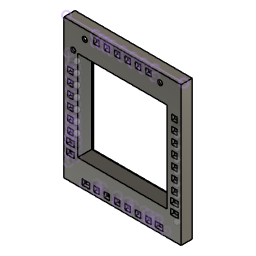
AH64-Iteration 6 v4 (Autodesk Fusion 360 design; units mm, degrees)
Autodesk Fusion 360 part; units mm, degrees
note: some values were not read from the file. Set by a fixed rule: which sketch regions a step uses.
(part 1 of 2)
sketch "Main Bezel" plane through (0, 0, 0) normal (0, 1, 0) x (1, 0, 0)
  line L0 (-54.051, 54.555) -> (-54.051, -54.555)
  line L1 (84.051, -99.755) -> (84.051, 99.755)
  line L2 (54.051, 54.555) -> (-54.051, 54.555)
  line L3 (-84.051, -99.755) -> (84.051, -99.755)
  line L4 (-54.051, -54.555) -> (54.051, -54.555)
  line L5 (-84.051, 99.755) -> (-84.051, -99.755)
  line L6 (84.051, 99.755) -> (-84.051, 99.755)
  line L7 (54.051, -54.555) -> (54.051, 54.555)
  point P0 (-27.075, -27.8271)
  dimension "d1" = 108.102
  dimension "d2" = 45.2
  dimension "d3" = 45.2
  dimension "d4" = 30
  dimension "d5" = 30
  dimension "d6" = 199.51
  dimension "d7" = 168.102
  dimension "d8" = 54.051
  dimension "d10" = 54.555
  dimension "d11" = 54.555
  dimension "d12" = 54.051
  constraint horizontal L4
  constraint vertical L7
  constraint horizontal L2
  constraint vertical L0
  constraint horizontal L3
  constraint vertical L1
  constraint horizontal L6
  constraint vertical L5
  measures "d1" distance of L0.end L4.end
  measures "d2" distance of L2 L6
  measures "d3" distance of L3 L4
  measures "d4" distance of L1 L7
  measures "d5" distance of L0 L5
  measures "d6" distance of L1.end L1.start
  measures "d7" distance of L3.start L1.start
  measures "d8" distance of origin L7
  measures "d10" distance of origin L4
  measures "d11" distance of origin L2
  measures "d12" distance of origin L0
extrude "Extrude1" add sketch "Main Bezel" along normal blind 16
sketch "LCD and Switch Insets" plane through (0, 16, 0) normal (0, 1, 0) x (-1, 0, 0)
  line L0 (-54.051, -54.555) -> (-54.051, 54.555)
  line L1 (-54.051, 54.555) -> (54.051, 54.555)
  line L2 (54.051, 54.555) -> (54.051, -54.555)
  line L3 (54.051, -54.555) -> (-54.051, -54.555)
  line L4 (-84.051, -99.755) -> (84.051, -99.755)
  line L5 (84.051, -99.755) -> (84.051, 99.755)
  line L6 (84.051, 99.755) -> (-84.051, 99.755)
  line L7 (-84.051, 99.755) -> (-84.051, -99.755)
  line L8 (-62.651, 73.5) -> (57.349, 73.5)
  line L9 (57.349, 73.5) -> (57.349, -81.5)
  line L10 (-62.651, -58.885) -> (-66.051, -58.885)
  line L11 (-66.051, -58.885) -> (-66.051, -8.885)
  line L12 (-66.051, -8.885) -> (-62.651, -8.885)
  line L13 (-52.651, -81.5) -> (-52.651, -84.7)
  line L14 (-52.651, -84.7) -> (-62.4877, -84.7)
  line L15 (-62.4877, -84.7) -> (-62.4877, -79.7)
  line L16 (-62.651, 73.5) -> (-62.651, -8.885)
  line L17 (-62.651, -58.885) -> (-62.4877, -79.7)
  line L18 (-52.651, -81.5) -> (57.349, -81.5)
  line L19 (-81.051, 62.605) -> (-68.051, 62.605)
  line L20 (-68.051, 62.605) -> (-68.051, -86.395)
  line L21 (-68.051, -86.395) -> (-81.051, -86.395)
  line L22 (-81.051, -86.395) -> (-81.051, 62.605)
  line L23 (68.051, 55.005) -> (81.051, 55.005)
  line L24 (81.051, 55.005) -> (81.051, -80.995)
  line L25 (81.051, -80.995) -> (68.051, -80.995)
  line L26 (68.051, -80.995) -> (68.051, 55.005)
  line L27 (-42.501, 96.755) -> (42.499, 96.755)
  line L28 (42.499, 96.755) -> (42.499, 86.755)
  line L29 (42.499, 86.755) -> (-42.501, 86.755)
  line L30 (-42.501, 86.755) -> (-42.501, 96.755)
  line L31 (-58.499, -86.755) -> (58.501, -86.755)
  line L32 (58.501, -86.755) -> (58.501, -96.755)
  line L33 (58.501, -96.755) -> (-58.499, -96.755)
  line L34 (-58.499, -96.755) -> (-58.499, -86.755)
  dimension "d15" = 120
  dimension "d18" = 3.298
  dimension "d19" = 18.945
  dimension "d21" = 3.4
  dimension "d22" = 50
  dimension "d23" = 10
  dimension "d24" = 5
  dimension "d25" = 13
  dimension "d27" = 37.15
  dimension "d28" = 3
  dimension "d29" = 13
  dimension "d30" = 136
  dimension "d31" = 3
  dimension "d32" = 44.75
  dimension "d33" = 85
  dimension "d34" = 10
  dimension "d35" = 3
  dimension "d36" = 41.55
  dimension "d37" = 117
  dimension "d38" = 10
  dimension "d39" = 3
  dimension "d40" = 25.55
  dimension "d108" = 149
  dimension "d109" = 13
  dimension "d170" = 3.2
  constraint horizontal L8
  constraint vertical L9
  constraint horizontal L10
  constraint vertical L11
  constraint horizontal L12
  constraint vertical L13
  constraint horizontal L14
  constraint vertical L15
  constraint perpendicular L12 L16
  constraint perpendicular L9 L18
  constraint horizontal L19
  constraint vertical L20
  constraint horizontal L21
  constraint vertical L22
  constraint horizontal L23
  constraint vertical L24
  constraint horizontal L25
  constraint vertical L26
  constraint horizontal L27
  constraint vertical L28
  constraint horizontal L29
  constraint vertical L30
  constraint horizontal L31
  constraint vertical L32
  constraint horizontal L33
  constraint vertical L34
  measures "d15" distance of L8.start L8.end
  measures "d18" distance of L2 L9
  measures "d19" distance of L1 L8
  measures "d21" distance of L10.start L10.end
  measures "d22" distance of L10.start L12.end
  measures "d23" distance of L15.end L13.start
  measures "d24" distance of L15.end L14.end
  measures "d25" distance of L19.start L19.end
  measures "d27" distance of L6 L19
  measures "d28" distance of L7 L22
  measures "d29" distance of L23.start L23.end
  measures "d30" distance of L23.start L25.end
  measures "d31" distance of L5 L24
  measures "d32" distance of L6 L23
  measures "d33" distance of L27.start L27.end
  measures "d34" distance of L27.start L29.end
  measures "d35" distance of L6 L27
  measures "d36" distance of L7 L30
  measures "d37" distance of L31.start L31.end
  measures "d38" distance of L31.start L33.end
  measures "d39" distance of L4 L33
  measures "d40" distance of L5 L32
  measures "d108" distance of L19.start L21.end
  measures "d109" distance of L20.end L21.end
  measures "d170" distance of L13.start L13.end
extrude "Extrude2" cut sketch "LCD and Switch Insets" against normal blind 5 contours L8 L9 L10 L11 L12 L13 L14 L15 L16 L17 L18
extrude "Extrude3" cut sketch "LCD and Switch Insets" against normal blind 12 contours L19 L20 L21 L22 | L23 L24 L25 L26 | L27 L28 L29 L30 | L31 L32 L33 L34
sketch "Button Holes" plane through (0, 16, 0) normal (0, 1, 0) x (-1, 0, 0)
  line L0 (-54.051, 54.5551) -> (-84.051, 54.5551) construction
  line L1 (-78.351, 41.5551) -> (-70.751, 41.5551)
  line L2 (-70.751, 41.5551) -> (-70.751, 33.9551)
  line L3 (-70.751, 33.9551) -> (-78.351, 33.9551)
  line L4 (-78.351, 33.9551) -> (-78.351, 41.5551)
  line L5 (-81.051, 62.605) -> (-68.051, 62.605)
  line L6 (-84.051, 99.755) -> (-84.051, -99.755)
  line L7 (-68.051, 62.605) -> (-68.051, -86.395)
  line L8 (-81.051, -86.395) -> (-81.051, 62.605)
  line L9 (84.051, 99.755) -> (-84.051, 99.755)
  line L10 (-78.351, 56.6551) -> (-70.751, 56.6551)
  line L11 (-70.751, 56.6551) -> (-70.751, 49.0551)
  line L12 (-70.751, 49.0551) -> (-78.351, 49.0551)
  line L13 (-78.351, 49.0551) -> (-78.351, 56.6551)
  line L14 (-78.351, -33.9474) -> (-70.751, -33.9474)
  line L15 (-70.751, -33.9474) -> (-70.751, -41.5474)
  line L16 (-70.751, -41.5474) -> (-78.351, -41.5474)
  line L17 (-78.351, -41.5474) -> (-78.351, -33.9474)
  line L18 (-54.051, -54.5474) -> (-84.051, -54.5474) construction
  line L19 (-84.051, -99.755) -> (84.051, -99.755)
  line L20 (-70.751, -26.4474) -> (-78.351, -26.4474)
  line L21 (-78.351, -26.4474) -> (-78.351, -18.8474)
  line L22 (-78.351, -18.8474) -> (-70.751, -18.8474)
  line L23 (-70.751, -18.8474) -> (-70.751, -26.4474)
  line L24 (-70.751, -11.3474) -> (-78.351, -11.3474)
  line L25 (-78.351, -11.3474) -> (-78.351, -3.7474)
  line L26 (-78.351, -3.7474) -> (-70.751, -3.7474)
  line L27 (-70.751, -3.7474) -> (-70.751, -11.3474)
  line L28 (-70.751, 3.7526) -> (-78.351, 3.7526)
  line L29 (-78.351, 3.7526) -> (-78.351, 11.3526)
  line L30 (-78.351, 11.3526) -> (-70.751, 11.3526)
  line L31 (-70.751, 11.3526) -> (-70.751, 3.7526)
  line L32 (-70.751, 18.8526) -> (-78.351, 18.8526)
  line L33 (-78.351, 18.8526) -> (-78.351, 26.4526)
  line L34 (-78.351, 26.4526) -> (-70.751, 26.4526)
  line L35 (-70.751, 26.4526) -> (-70.751, 18.8526)
  line L36 (-79.851, -47.5474) -> (-69.251, -47.5474)
  line L37 (-69.251, -47.5474) -> (-69.251, -55.1474)
  line L38 (-69.251, -55.1474) -> (-79.851, -55.1474)
  line L39 (-79.851, -55.1474) -> (-79.851, -47.5474)
  line L40 (-79.851, -61.1474) -> (-69.251, -61.1474)
  line L41 (-69.251, -61.1474) -> (-69.251, -68.7474)
  line L42 (-69.251, -68.7474) -> (-79.851, -68.7474)
  line L43 (-79.851, -68.7474) -> (-79.851, -61.1474)
  line L44 (78.351, 33.9551) -> (70.751, 33.9551)
  line L45 (70.751, 33.9551) -> (70.751, 41.5551)
  line L46 (70.751, 41.5551) -> (78.351, 41.5551)
  line L47 (78.351, 41.5551) -> (78.351, 33.9551)
  line L48 (70.751, 18.8526) -> (70.751, 26.4526)
  line L49 (70.751, 26.4526) -> (78.351, 26.4526)
  line L50 (78.351, 18.8526) -> (70.751, 18.8526)
  line L51 (78.351, 26.4526) -> (78.351, 18.8526)
  line L52 (70.751, 3.7526) -> (70.751, 11.3526)
  line L53 (70.751, 11.3526) -> (78.351, 11.3526)
  line L54 (78.351, 3.7526) -> (70.751, 3.7526)
  line L55 (78.351, 11.3526) -> (78.351, 3.7526)
  line L56 (70.751, -11.3474) -> (70.751, -3.7474)
  line L57 (70.751, -3.7474) -> (78.351, -3.7474)
  line L58 (78.351, -11.3474) -> (70.751, -11.3474)
  line L59 (78.351, -3.7474) -> (78.351, -11.3474)
  line L60 (70.751, -26.4474) -> (70.751, -18.8474)
  line L61 (70.751, -18.8474) -> (78.351, -18.8474)
  line L62 (78.351, -26.4474) -> (70.751, -26.4474)
  line L63 (78.351, -18.8474) -> (78.351, -26.4474)
  line L64 (70.751, -41.5474) -> (70.751, -33.9474)
  line L65 (70.751, -33.9474) -> (78.351, -33.9474)
  line L66 (78.351, -41.5474) -> (70.751, -41.5474)
  line L67 (78.351, -33.9474) -> (78.351, -41.5474)
  line L68 (84.051, -99.755) -> (84.051, 99.755)
  line L69 (68.051, -80.995) -> (68.051, 55.005)
  line L70 (69.251, -68.7474) -> (69.251, -61.1474)
  line L71 (69.251, -61.1474) -> (79.851, -61.1474)
  line L72 (79.851, -61.1474) -> (79.851, -68.7474)
  line L73 (79.851, -68.7474) -> (69.251, -68.7474)
  line L74 (79.851, -55.1474) -> (69.251, -55.1474)
  line L75 (69.251, -55.1474) -> (69.251, -47.5474)
  line L76 (79.851, -47.5474) -> (79.851, -55.1474)
  line L77 (69.251, -47.5474) -> (79.851, -47.5474)
  line L78 (-54.051, -54.5474) -> (-54.051, -99.755) construction
  line L79 (-41.051, -87.955) -> (-33.451, -87.955)
  line L80 (-33.451, -87.955) -> (-33.451, -95.555)
  line L81 (-33.451, -95.555) -> (-41.051, -95.555)
  line L82 (-41.051, -95.555) -> (-41.051, -87.955)
  line L83 (58.501, -86.755) -> (58.501, -96.755)
  line L84 (58.501, -96.755) -> (-58.499, -96.755)
  line L85 (-26.151, -95.555) -> (-26.151, -87.955)
  line L86 (-26.151, -87.955) -> (-18.551, -87.955)
  line L87 (-18.551, -87.955) -> (-18.551, -95.555)
  line L88 (-18.551, -95.555) -> (-26.151, -95.555)
  line L89 (-11.251, -95.555) -> (-11.251, -87.955)
  line L90 (-11.251, -87.955) -> (-3.651, -87.955)
  line L91 (-3.651, -87.955) -> (-3.651, -95.555)
  line L92 (-3.651, -95.555) -> (-11.251, -95.555)
  line L93 (3.649, -95.555) -> (3.649, -87.955)
  line L94 (3.649, -87.955) -> (11.249, -87.955)
  line L95 (11.249, -87.955) -> (11.249, -95.555)
  line L96 (11.249, -95.555) -> (3.649, -95.555)
  line L97 (18.549, -95.555) -> (18.549, -87.955)
  line L98 (18.549, -87.955) -> (26.149, -87.955)
  line L99 (26.149, -87.955) -> (26.149, -95.555)
  line L100 (26.149, -95.555) -> (18.549, -95.555)
  line L101 (33.451, -95.555) -> (33.451, -87.955)
  line L102 (33.451, -87.955) -> (41.051, -87.955)
  line L103 (41.051, -87.955) -> (41.051, -95.555)
  line L104 (41.051, -95.555) -> (33.451, -95.555)
  line L105 (54.051, -54.8879) -> (54.051, -99.755) construction
  line L106 (-57.651, -87.955) -> (-47.051, -87.955)
  line L107 (-47.051, -87.955) -> (-47.051, -95.555)
  line L108 (-47.051, -95.555) -> (-57.651, -95.555)
  line L109 (-57.651, -95.555) -> (-57.651, -87.955)
  line L110 (47.051, -87.955) -> (57.651, -87.955)
  line L111 (57.651, -87.955) -> (57.651, -95.555)
  line L112 (57.651, -95.555) -> (47.051, -95.555)
  line L113 (47.051, -95.555) -> (47.051, -87.955)
  line L114 (-33.451, 87.955) -> (-41.051, 87.955)
  line L115 (-41.051, 87.955) -> (-41.051, 95.555)
  line L116 (-41.051, 95.555) -> (-33.451, 95.555)
  line L117 (-33.451, 95.555) -> (-33.451, 87.955)
  line L118 (-26.151, 95.555) -> (-18.551, 95.555)
  line L119 (-18.551, 95.555) -> (-18.551, 87.955)
  line L120 (-26.151, 87.955) -> (-26.151, 95.555)
  line L121 (-18.551, 87.955) -> (-26.151, 87.955)
  line L122 (-11.251, 95.555) -> (-3.651, 95.555)
  line L123 (-3.651, 95.555) -> (-3.651, 87.955)
  line L124 (-11.251, 87.955) -> (-11.251, 95.555)
  line L125 (-3.651, 87.955) -> (-11.251, 87.955)
  line L126 (3.649, 95.555) -> (11.249, 95.555)
  line L127 (11.249, 95.555) -> (11.249, 87.955)
  line L128 (3.649, 87.955) -> (3.649, 95.555)
  line L129 (11.249, 87.955) -> (3.649, 87.955)
  line L130 (18.549, 95.555) -> (26.149, 95.555)
  line L131 (26.149, 95.555) -> (26.149, 87.955)
  line L132 (18.549, 87.955) -> (18.549, 95.555)
  line L133 (26.149, 87.955) -> (18.549, 87.955)
  line L134 (33.451, 95.555) -> (41.051, 95.555)
  line L135 (41.051, 95.555) -> (41.051, 87.955)
  line L136 (33.451, 87.955) -> (33.451, 95.555)
  line L137 (41.051, 87.955) -> (33.451, 87.955)
  line L138 (42.499, 96.755) -> (42.499, 86.755)
  line L139 (-58.499, -86.755) -> (58.501, -86.755)
  line L140 (-42.501, 96.755) -> (42.499, 96.755)
  line L141 (42.499, 86.755) -> (-42.501, 86.755)
  dimension "d45" = 7.6
  dimension "d46" = 7.6
  dimension "d47" = 13
  dimension "d48" = 5.7
  dimension "d49" = 2.7
  dimension "d50" = 2.7
  dimension "d51" = 30
  dimension "d52" = 45.1999
  dimension "d54" = 13
  dimension "d55" = 7.6
  dimension "d56" = 7.6
  dimension "d57" = 7.5
  dimension "d66" = 5.7
  dimension "d74" = 7.6
  dimension "d75" = 7.6
  dimension "d78" = 5.7
  dimension "d79" = 13
  dimension "d80" = 45.2076
  dimension "d81" = 30
  dimension "d82" = 67.9024
  dimension "d83" = 7.6
  dimension "d84" = 7.6
  dimension "d85" = 7.6
  dimension "d86" = 7.6
  dimension "d87" = 7.6
  dimension "d88" = 7.6
  dimension "d89" = 7.6
  dimension "d90" = 7.6
  dimension "d91" = 7.5
  dimension "d92" = 7.5
  dimension "d93" = 7.5
  dimension "d94" = 7.5
  dimension "d95" = 7.5024
  dimension "d96" = 5.7
  dimension "d97" = 5.7
  dimension "d98" = 5.7
  dimension "d99" = 5.7
  dimension "d100" = 10.6
  dimension "d101" = 7.6
  dimension "d102" = 4.2
  dimension "d103" = 6
  dimension "d104" = 10.6
  dimension "d105" = 7.6
  dimension "d106" = 6
  dimension "d107" = 4.2
  dimension "d112" = 7.6
  dimension "d113" = 7.6
  dimension "d114" = 7.6
  dimension "d115" = 7.6
  dimension "d116" = 67.9024
  dimension "d117" = 7.6
  dimension "d118" = 7.6
  dimension "d119" = 7.6
  dimension "d120" = 7.6
  dimension "d121" = 7.6
  dimension "d122" = 7.6
  dimension "d123" = 7.6
  dimension "d124" = 7.6
  dimension "d125" = 7.5
  dimension "d126" = 7.5
  dimension "d127" = 7.5
  dimension "d128" = 7.5
  dimension "d129" = 7.5024
  dimension "d130" = 5.7
  dimension "d131" = 2.7
  dimension "d132" = 5.7
  dimension "d133" = 5.7
  dimension "d134" = 58.2076
  dimension "d135" = 58.2076
  dimension "d136" = 10.6
  dimension "d137" = 7.6
  dimension "d138" = 10.6
  dimension "d139" = 7.6
  dimension "d140" = 6
  dimension "d141" = 4.2
  dimension "d142" = 31.0076
  dimension "d143" = 31.0076
  dimension "d144" = 7.6
  dimension "d145" = 7.6
  dimension "d146" = 13
  dimension "d147" = 10
  dimension "d148" = 3
  dimension "d149" = 4.2
  dimension "d150" = 7.6
  dimension "d151" = 7.6
  dimension "d152" = 7.6
  dimension "d153" = 7.6
  dimension "d154" = 7.6
  dimension "d155" = 7.6
  dimension "d156" = 7.6
  dimension "d157" = 7.6
  dimension "d158" = 7.6
  dimension "d159" = 7.6
  dimension "d160" = 13
  dimension "d161" = 30
  dimension "d162" = 30
  dimension "d163" = 7.3
  dimension "d164" = 7.3
  dimension "d165" = 7.3
  dimension "d166" = 7.3
  dimension "d167" = 7.302
  dimension "d168" = 10.6
  dimension "d169" = 7.6
  dimension "d171" = 6
  dimension "d172" = 10.6
  dimension "d173" = 7.6
  dimension "d174" = 6
  dimension "d176" = 4.2
  dimension "d177" = 7.6
  dimension "d178" = 7.6
  dimension "d179" = 7.6
  dimension "d180" = 7.6
  dimension "d181" = 7.6
  dimension "d182" = 7.6
  dimension "d183" = 7.6
  dimension "d184" = 7.6
  dimension "d185" = 7.6
  dimension "d186" = 7.6
  dimension "d187" = 7.6
  dimension "d188" = 7.6
  dimension "d189" = 7.3
  dimension "d190" = 7.3
  dimension "d191" = 7.3
  dimension "d192" = 7.3
  dimension "d193" = 7.302
  dimension "d194" = 4.2
  dimension "d195" = 4.2
  dimension "d196" = 4.2
  dimension "d197" = 4.2
  dimension "d198" = 4.2
  dimension "d199" = 43
  dimension "d200" = 1.448
  dimension "d201" = 43
  dimension "d202" = 7.6
  dimension "d203" = 4.2
  dimension "d224" = 1.2
  dimension "d225" = 1.2
  dimension "d226" = 2.7
  dimension "d227" = 7.6
  dimension "d228" = 5.7
  dimension "d229" = 5.7
  dimension "d230" = 5.7
  dimension "d232" = 4.2
  dimension "d234" = 1.2
  dimension "d235" = 1.2
  dimension "d236" = 4.2
  dimension "d237" = 4.2
  dimension "d238" = 4.2
  dimension "d239" = 4.2
  dimension "d240" = 4.2
  dimension "d242" = 4.2
  dimension "d243" = 1.2
  dimension "d244" = 1.2
  constraint horizontal L0
  constraint horizontal L1
  constraint vertical L2
  constraint horizontal L3
  constraint vertical L4
  constraint horizontal L10
  constraint vertical L11
  constraint horizontal L12
  constraint vertical L13
  constraint horizontal L14
  constraint vertical L15
  constraint horizontal L16
  constraint vertical L17
  constraint coincident L6 L18.end
  constraint perpendicular L6 L18
  constraint horizontal L22
  constraint vertical L23
  constraint horizontal L20
  constraint vertical L21
  constraint horizontal L26
  constraint vertical L27
  constraint horizontal L24
  constraint vertical L25
  constraint horizontal L30
  constraint vertical L31
  constraint horizontal L28
  constraint vertical L29
  constraint horizontal L34
  constraint vertical L35
  constraint horizontal L32
  constraint vertical L33
  constraint horizontal L36
  constraint vertical L37
  constraint horizontal L38
  constraint vertical L39
  constraint horizontal L40
  constraint vertical L41
  constraint horizontal L42
  constraint vertical L43
  constraint horizontal L46
  constraint vertical L47
  constraint horizontal L44
  constraint vertical L45
  constraint horizontal L65
  constraint vertical L67
  constraint horizontal L66
  constraint vertical L64
  constraint horizontal L61
  constraint vertical L63
  constraint horizontal L62
  constraint vertical L60
  constraint horizontal L57
  constraint vertical L59
  constraint horizontal L58
  constraint vertical L56
  constraint horizontal L53
  constraint vertical L55
  constraint horizontal L54
  constraint vertical L52
  constraint horizontal L49
  constraint vertical L51
  constraint horizontal L50
  constraint vertical L48
  constraint horizontal L77
  constraint vertical L76
  constraint horizontal L74
  constraint vertical L75
  constraint horizontal L71
  constraint vertical L72
  constraint horizontal L73
  constraint vertical L70
  constraint coincident L19 L78.end
  constraint perpendicular L19 L78
  constraint horizontal L79
  constraint vertical L80
  constraint horizontal L81
  constraint vertical L82
  constraint horizontal L86
  constraint vertical L87
  constraint horizontal L88
  constraint vertical L85
  constraint horizontal L90
  constraint vertical L91
  constraint horizontal L92
  constraint vertical L89
  constraint horizontal L94
  constraint vertical L95
  constraint horizontal L96
  constraint vertical L93
  constraint horizontal L98
  constraint vertical L99
  constraint horizontal L100
  constraint vertical L97
  constraint horizontal L102
  constraint vertical L103
  constraint horizontal L104
  constraint vertical L101
  constraint coincident L19 L105.end
  constraint perpendicular L19 L105
  constraint horizontal L106
  constraint vertical L107
  constraint horizontal L108
  constraint vertical L109
  constraint horizontal L110
  constraint vertical L111
  constraint horizontal L112
  constraint vertical L113
  constraint horizontal L116
  constraint vertical L117
  constraint horizontal L114
  constraint vertical L115
  constraint horizontal L118
  constraint vertical L119
  constraint horizontal L121
  constraint vertical L120
  constraint horizontal L122
  constraint vertical L123
  constraint horizontal L125
  constraint vertical L124
  constraint horizontal L126
  constraint vertical L127
  constraint horizontal L129
  constraint vertical L128
  constraint horizontal L130
  constraint vertical L131
  constraint horizontal L133
  constraint vertical L132
  constraint horizontal L134
  constraint vertical L135
  constraint horizontal L137
  constraint vertical L136
  measures "d45" distance of L1.start L1.end
  measures "d46" distance of L1.start L3.end
  measures "d47" distance of L5.start L5.end
  measures "d48" distance of L4 L6
  measures "d49" distance of L2 L7
  measures "d50" distance of L4 L8
  measures "d51" distance of L0.start L0.end
  measures "d52" distance of L0 L9
  measures "d54" distance of L0 L1
  measures "d55" distance of L10.end L10.start
  measures "d56" distance of L12.end L10.start
  measures "d57" distance of L1 L12
  measures "d66" distance of L6 L13
  measures "d74" distance of L14.end L14.start
  measures "d75" distance of L14.start L16.end
  measures "d78" distance of L6 L17
  measures "d79" distance of L16 L18
  measures "d80" distance of L18 L19
  measures "d81" distance of L6 L18.start
  measures "d82" distance of L3 L14
  measures "d83" distance of L22.end L21.end
  measures "d84" distance of L20.end L21.end
  measures "d85" distance of L26.end L25.end
  measures "d86" distance of L24.end L25.end
  measures "d87" distance of L30.end L29.end
  measures "d88" distance of L28.end L29.end
  measures "d89" distance of L34.end L33.end
  measures "d90" distance of L32.end L33.end
  measures "d91" distance of L14 L20
  measures "d92" distance of L22 L24
  measures "d93" distance of L26 L28
  measures "d94" distance of L30 L32
  measures "d95" distance of L3 L34
  measures "d96" distance of L6 L33
  measures "d97" distance of L6 L29
  measures "d98" distance of L6 L25
  measures "d99" distance of L6 L21
  measures "d100" distance of L36.start L36.end
  measures "d101" distance of L36.start L38.end
  measures "d102" distance of L6 L39
  measures "d103" distance of L16 L36
  measures "d104" distance of L40.start L40.end
  measures "d105" distance of L40.start L42.end
  measures "d106" distance of L38 L40
  measures "d107" distance of L6 L43
  measures "d112" distance of L46.end L45.end
  measures "d113" distance of L44.end L45.end
  measures "d114" distance of L65.end L64.end
  measures "d115" distance of L64.start L64.end
  measures "d116" distance of L44 L65
  measures "d117" distance of L60.end L61.end
  measures "d118" distance of L60.end L60.start
  measures "d119" distance of L57.end L56.end
  measures "d120" distance of L56.start L56.end
  measures "d121" distance of L52.end L53.end
  measures "d122" distance of L52.end L52.start
  measures "d123" distance of L49.end L48.end
  measures "d124" distance of L48.start L48.end
  measures "d125" distance of L62 L65
  measures "d126" distance of L58 L61
  measures "d127" distance of L54 L57
  measures "d128" distance of L50 L53
  measures "d129" distance of L44 L49
  measures "d130" distance of L47 L68
  measures "d131" distance of L45 L69
  measures "d132" distance of L51 L68
  measures "d133" distance of L67 L68
  measures "d134" distance of L19 L66
  measures "d135" distance of L16 L19
  measures "d136" distance of L75.end L76.start
  measures "d137" distance of L75.end L74.end
  measures "d138" distance of L70.end L71.end
  measures "d139" distance of L70.end L70.start
  measures "d140" distance of L71 L74
  measures "d141" distance of L68 L72
  measures "d142" distance of L19 L42
  measures "d143" distance of L19 L73
  measures "d144" distance of L79.start L79.end
  measures "d145" distance of L79.start L81.end
  measures "d146" distance of L78 L82
  measures "d147" distance of L83.start L83.end
  measures "d148" distance of L19 L84
  measures "d149" distance of L19 L81
  measures "d150" distance of L86.end L85.end
  measures "d151" distance of L85.start L85.end
  measures "d152" distance of L90.end L89.end
  measures "d153" distance of L89.start L89.end
  measures "d154" distance of L94.end L93.end
  measures "d155" distance of L93.start L93.end
  measures "d156" distance of L98.end L97.end
  measures "d157" distance of L97.start L97.end
  measures "d158" distance of L102.end L101.end
  measures "d159" distance of L101.start L101.end
  measures "d160" distance of L103 L105
  measures "d161" distance of L68 L105
  measures "d162" distance of L6 L78
  measures "d163" distance of L80 L85
  measures "d164" distance of L87 L89.start
  measures "d165" distance of L91 L93
  measures "d166" distance of L95 L97
  measures "d167" distance of L99 L101
  measures "d168" distance of L106.start L106.end
  measures "d169" distance of L106.start L108.end
  measures "d171" distance of L82 L107
  measures "d172" distance of L110.end L110.start
  measures "d173" distance of L110.start L112.end
  measures "d174" distance of L103 L113
  measures "d176" distance of L19 L108
  measures "d177" distance of L116.end L115.end
  measures "d178" distance of L114.end L115.end
  measures "d179" distance of L118.end L118.start
  measures "d180" distance of L120.start L118.start
  measures "d181" distance of L122.end L122.start
  measures "d182" distance of L122.start L124.start
  measures "d183" distance of L126.end L126.start
  measures "d184" distance of L126.start L128.start
  measures "d185" distance of L130.end L130.start
  measures "d186" distance of L132.start L130.start
  measures "d187" distance of L134.start L134.end
  measures "d188" distance of L134.start L136.start
  measures "d189" distance of L117 L120
  measures "d190" distance of L124.start L119
  measures "d191" distance of L123 L128
  measures "d192" distance of L127 L132
  measures "d193" distance of L131 L136
  measures "d194" distance of L9 L116
  measures "d195" distance of L9 L134
  measures "d196" distance of L9 L130
  measures "d197" distance of L9 L122
  measures "d198" distance of L9 L126
  measures "d199" distance of L6 L115
  measures "d200" distance of L135 L138
  measures "d201" distance of L68 L135
  measures "d202" distance of L118.end L118.start
  measures "d203" distance of L9 L118
  measures "d224" distance of L8 L43
  measures "d225" distance of L7 L41
  measures "d226" distance of L4 L8
  measures "d227" distance of L54.start L53.end
  measures "d228" distance of L55 L68
  measures "d229" distance of L59 L68
  measures "d230" distance of L63 L68
  measures "d232" distance of L68 L76
  measures "d234" distance of L81 L84
  measures "d235" distance of L79 L139
  measures "d236" distance of L19 L88
  measures "d237" distance of L19 L92
  measures "d238" distance of L19 L96
  measures "d239" distance of L19 L100
  measures "d240" distance of L19 L104
  measures "d242" distance of L19 L112
  measures "d243" distance of L130 L140
  measures "d244" distance of L133 L141
chamfer "Chamfer1" distance 10 angle 45 2 edges at (54.051, 0, 0) (-54.051, 0, 0)
chamfer "Chamfer2" distance 10 angle 45 2 edges at (0, 0, -54.555) (0, 0, 54.555)
extrude "Extrude4" cut sketch "Button Holes" against normal through all contours L1 L2 L3 L4 | L10 L11 L12 L13 | L14 L15 L16 L17 | L20 L21 L22 L23 | L24 L25 L26 L27 | L28 L29 L30 L31 | L32 L33 L34 L35 | L36 L37 L38 L39 | L40 L41 L42 L43 | L44 L45 L46 L47 | L48 L49 L50 L51 | L52 L53 L54 L55 | L56 L57 L58 L59 | L60 L61 L62 L63 | L64 L65 L66 L67 | L70 L71 L72 L73 | L74 L75 L76 L77 | L79 L80 L81 L82 | L85 L86 L87 L88 | L89 L90 L91 L92 | L93 L94 L95 L96 | L97 L98 L99 L100 | L101 L102 L103 L104 | L106 L107 L108 L109 | L110 L111 L112 L113 | L114 L115 L116 L117 | L118 L119 L120 L121 | L122 L123 L124 L125 | L126 L127 L128 L129 | L130 L131 L132 L133 | L134 L135 L136 L137
sketch "Pot Holes" plane through (0, 16, 0) normal (0, 1, 0) x (-1, 0, 0)
  line L0 (-68.051, 62.605) -> (-68.051, -86.395)
  line L1 (-66.051, -8.885) -> (-62.651, -8.885)
  line L2 (-62.651, -8.885) -> (-62.651, 73.5)
  line L3 (-62.651, 73.5) -> (57.349, 73.5)
  line L4 (57.349, 73.5) -> (57.349, -81.5)
  line L5 (57.349, -81.5) -> (-52.651, -81.5)
  line L6 (-52.651, -81.5) -> (-52.651, -84.7)
  line L7 (-52.651, -84.7) -> (-62.4877, -84.7)
  line L8 (-62.4877, -84.7) -> (-62.4877, -79.7)
  line L9 (-62.4877, -79.7) -> (-62.651, -58.885)
  line L10 (-62.651, -58.885) -> (-66.051, -58.885)
  line L11 (-68.051, -86.395) -> (-81.051, -86.395)
  line L12 (-81.051, -86.395) -> (-81.051, 62.605)
  line L13 (-81.051, 62.605) -> (-68.051, 62.605)
  line L14 (42.499, 96.755) -> (42.499, 86.755)
  line L15 (42.499, 86.755) -> (-42.501, 86.755)
  line L16 (-42.501, 86.755) -> (-42.501, 96.755)
  line L17 (-42.501, 96.755) -> (42.499, 96.755)
  line L18 (58.501, -86.755) -> (58.501, -96.755)
  line L19 (58.501, -96.755) -> (-58.499, -96.755)
  line L20 (-58.499, -96.755) -> (-58.499, -86.755)
  line L21 (-58.499, -86.755) -> (58.501, -86.755)
  line L22 (81.051, 55.005) -> (81.051, -80.995)
  line L23 (81.051, -80.995) -> (68.051, -80.995)
  line L24 (68.051, -80.995) -> (68.051, 55.005)
  line L25 (68.051, 55.005) -> (81.051, 55.005)
  line L26 (-84.051, -99.755) -> (84.051, -99.755)
  line L27 (84.051, -99.755) -> (84.051, 99.755)
  line L28 (84.051, 99.755) -> (-84.051, 99.755)
  line L29 (-84.051, 99.755) -> (-84.051, -99.755)
  line L30 (-61.1795, 95.8145) -> (-53.6199, 95.4435)
  line L31 (-61.1795, 95.8145) -> (-70.0401, 95.755)
  line L32 (-70.0401, 95.755) -> (-70.0334, 77.755)
  line L33 (-70.0334, 77.755) -> (-61.0335, 77.7955)
  line L34 (-61.0335, 77.7955) -> (-53.3792, 78.4668)
  arc A0 (-53.3792, 78.4668) -> (-53.6199, 95.4435) centre (-54.0368, 86.9476) ccw
  circle A1 centre (-53.8955, 87.2951) radius 3.5
  line L35 (61.7577, 77.7396) -> (54.2009, 78.164)
  line L36 (70.0689, 95.7955) -> (61.069, 95.755)
  line L37 (61.069, 95.755) -> (54.0803, 95.142)
  arc A2 (54.0803, 95.142) -> (54.2009, 78.164) centre (54.6779, 86.6568) ccw
  circle A3 centre (53.896, 86.9818) radius 3.5
  line L38 (61.792, 72.6199) -> (62.4634, 64.9657)
  arc A4 (62.4634, 64.9657) -> (79.4401, 65.2063) centre (70.9441, 65.6232) ccw
  line L39 (79.811, 72.7659) -> (79.4401, 65.2063)
  line L40 (79.811, 72.7659) -> (79.7516, 81.6265)
  circle A5 centre (70.5652, 65.4469) radius 3.5
  line L41 (61.792, 72.6199) -> (61.7577, 77.7396)
  line L42 (70.0689, 95.7955) -> (70.0742, 81.6229)
  line L43 (70.0742, 81.6229) -> (79.7516, 81.6265)
  line L44 (-66.051, -58.885) -> (-66.051, -8.885)
  dimension "d205" = 9
  dimension "d206" = 18
  dimension "d207" = 16
  dimension "d208" = 4
  dimension "d209" = 30.1555
  dimension "d210" = 9
  dimension "d214" = 179.742
  dimension "d215" = 4
  dimension "d216" = 30.155
  dimension "d220" = 6.1164
  constraint tangent L30 A0
  constraint tangent L35 A2
  constraint tangent A4 L39
  constraint coincident L35.start L41.end
  measures "d205" distance of L32.end L33.end
  measures "d206" distance of L32.end L31.end
  measures "d207" distance of A0.centre L32
  measures "d208" distance of L28 L31.end
  measures "d209" distance of L29 A1.centre
  measures "d210" distance of L36.start L36.end
  measures "d214" angle of L28 L36
  measures "d215" distance of L28 L36.end
  measures "d216" distance of L27 A3.centre
  measures "d220" distance of L3.end L35.start
extrude "Extrude5" cut sketch "Pot Holes" against normal blind 14 contours L30 L31 L32 L33 L34 A0 | L35 L36 L37 A2 L38 A4 L39 L40 L41 L42 L43
extrude "Extrude6" cut 3 faces at (55.7119, 16, 86.6379) (-54.1556, 16, 85.8444) (-71.6801, 16, 65.103) along direction (0, -1, 0) through all
sketch "Switch Screw Holes" plane through (0, 4, 0) normal (0, 1, 0) x (-1, 0, 0)
  line L0 (-79.851, -68.7474) -> (-79.851, -61.1474)
  line L1 (-79.851, -61.1474) -> (-69.251, -61.1474)
  line L2 (-69.251, -61.1474) -> (-69.251, -68.7474)
  line L3 (-69.251, -68.7474) -> (-79.851, -68.7474)
  line L4 (-70.751, -3.7474) -> (-70.751, -11.3474)
  line L5 (-70.751, -11.3474) -> (-78.351, -11.3474)
  line L6 (-78.351, -11.3474) -> (-78.351, -3.7474)
  line L7 (-78.351, -3.7474) -> (-70.751, -3.7474)
  line L8 (-78.351, 49.0551) -> (-78.351, 56.6551)
  line L9 (-78.351, 56.6551) -> (-70.751, 56.6551)
  line L10 (-70.751, 56.6551) -> (-70.751, 49.0551)
  line L11 (-70.751, 49.0551) -> (-78.351, 49.0551)
  line L12 (-70.751, 11.3526) -> (-70.751, 3.7526)
  line L13 (-70.751, 3.7526) -> (-78.351, 3.7526)
  line L14 (-78.351, 3.7526) -> (-78.351, 11.3526)
  line L15 (-78.351, 11.3526) -> (-70.751, 11.3526)
  line L16 (-79.851, -55.1474) -> (-79.851, -47.5474)
  line L17 (-79.851, -47.5474) -> (-69.251, -47.5474)
  line L18 (-69.251, -47.5474) -> (-69.251, -55.1474)
  line L19 (-69.251, -55.1474) -> (-79.851, -55.1474)
  line L20 (-70.751, -18.8474) -> (-70.751, -26.4474)
  line L21 (-70.751, -26.4474) -> (-78.351, -26.4474)
  line L22 (-78.351, -26.4474) -> (-78.351, -18.8474)
  line L23 (-78.351, -18.8474) -> (-70.751, -18.8474)
  line L24 (-78.351, 33.9551) -> (-78.351, 41.5551)
  line L25 (-78.351, 41.5551) -> (-70.751, 41.5551)
  line L26 (-70.751, 41.5551) -> (-70.751, 33.9551)
  line L27 (-70.751, 33.9551) -> (-78.351, 33.9551)
  line L28 (-70.751, 26.4526) -> (-70.751, 18.8526)
  line L29 (-70.751, 18.8526) -> (-78.351, 18.8526)
  line L30 (-78.351, 18.8526) -> (-78.351, 26.4526)
  line L31 (-78.351, 26.4526) -> (-70.751, 26.4526)
  line L32 (-78.351, -41.5474) -> (-78.351, -33.9474)
  line L33 (-78.351, -33.9474) -> (-70.751, -33.9474)
  line L34 (-70.751, -33.9474) -> (-70.751, -41.5474)
  line L35 (-70.751, -41.5474) -> (-78.351, -41.5474)
  line L36 (-81.051, -86.395) -> (-68.051, -86.395)
  line L37 (-68.051, -86.395) -> (-68.051, 62.605)
  line L38 (-68.051, 62.605) -> (-81.051, 62.605)
  line L39 (-81.051, 62.605) -> (-81.051, -86.395)
  line L40 (42.499, 86.755) -> (-42.501, 86.755)
  line L41 (-42.501, 96.755) -> (42.499, 96.755)
  line L42 (84.051, 99.755) -> (-84.051, 99.755)
  line L43 (33.451, 87.955) -> (33.451, 95.555)
  line L44 (26.149, 95.555) -> (26.149, 87.955)
  line L45 (18.549, 87.955) -> (18.549, 95.555)
  line L46 (3.649, 87.955) -> (3.649, 95.555)
  line L47 (-11.251, 87.955) -> (-11.251, 95.555)
  line L48 (-26.151, 87.955) -> (-26.151, 95.555)
  line L49 (-47.051, -87.955) -> (-47.051, -95.555)
  line L50 (-41.051, -95.555) -> (-41.051, -87.955)
  line L51 (-26.151, -95.555) -> (-26.151, -87.955)
  line L52 (-33.451, -87.955) -> (-33.451, -95.555)
  line L53 (58.501, -96.755) -> (-58.499, -96.755)
  line L54 (-11.251, -95.555) -> (-11.251, -87.955)
  line L55 (-3.651, -87.955) -> (-3.651, -95.555)
  line L56 (11.249, -87.955) -> (11.249, -95.555)
  line L57 (33.451, -95.555) -> (33.451, -87.955)
  line L58 (41.051, -87.955) -> (41.051, -95.555)
  line L59 (79.851, -68.7474) -> (69.251, -68.7474)
  line L60 (81.051, 55.005) -> (81.051, -80.995)
  line L61 (79.851, -55.1474) -> (69.251, -55.1474)
  line L62 (69.251, -47.5474) -> (79.851, -47.5474)
  line L63 (78.351, -41.5474) -> (70.751, -41.5474)
  line L64 (70.751, -33.9474) -> (78.351, -33.9474)
  line L65 (78.351, -26.4474) -> (70.751, -26.4474)
  line L66 (70.751, -18.8474) -> (78.351, -18.8474)
  line L67 (70.751, -3.7474) -> (78.351, -3.7474)
  line L68 (70.751, 11.3526) -> (78.351, 11.3526)
  line L69 (70.751, 26.4526) -> (78.351, 26.4526)
  line L70 (70.751, 41.5551) -> (78.351, 41.5551)
  point P0 (-74.551, 45.3051)
  point P1 (-74.551, 15.1026)
  point P2 (-74.551, 30.2026)
  point P3 (-74.551, 0.0026)
  point P4 (-74.551, -15.0974)
  point P5 (-74.551, -30.1974)
  point P6 (-74.551, -44.5474)
  point P7 (-74.551, -58.1474)
  point P8 (-74.551, -76.7825)
  point P9 (-44.051, -91.755)
  point P10 (-29.801, -91.755)
  point P11 (-14.901, -91.755)
  point P12 (-0.001, -91.755)
  point P13 (14.899, -91.755)
  point P14 (29.801, -91.755)
  point P15 (44.701, -91.755)
  point P16 (74.551, -73.7474)
  point P17 (74.551, -58.1474)
  point P18 (74.551, -44.5474)
  point P19 (74.551, -30.1974)
  point P20 (74.551, -15.0974)
  point P21 (74.551, 0.0026)
  point P22 (74.551, 15.1026)
  point P23 (74.551, 30.2026)
  point P24 (74.551, 46.5551)
  point P25 (29.801, 91.755)
  point P26 (14.899, 91.755)
  point P27 (-0.001, 91.755)
  point P28 (-14.901, 91.755)
  point P29 (-29.801, 91.755)
  dimension "d245" = 6.5
  dimension "d246" = 3
  dimension "d247" = 6
  dimension "d248" = 3
  dimension "d249" = 7.5
  dimension "d250" = 3.75
  dimension "d251" = 3.75
  dimension "d252" = 3.75
  dimension "d253" = 3.75
  dimension "d254" = 3.75
  dimension "d255" = 3.75
  dimension "d256" = 5
  dimension "d257" = 5
  dimension "d258" = 5
  dimension "d259" = 8
  dimension "d260" = 8
  dimension "d261" = 8
  dimension "d262" = 7.302
  dimension "d263" = 3.65
  dimension "d264" = 3.65
  dimension "d265" = 3.65
  dimension "d266" = 3.65
  dimension "d267" = 3.65
  dimension "d268" = 3
  dimension "d269" = 3
  dimension "d270" = 3.65
  dimension "d271" = 3.65
  dimension "d272" = 5
  dimension "d273" = 5
  dimension "d274" = 5
  dimension "d275" = 3.65
  dimension "d276" = 3.65
  dimension "d277" = 5
  dimension "d278" = 5
  dimension "d279" = 3.65
  dimension "d280" = 3.65
  dimension "d281" = 5
  dimension "d282" = 5
  dimension "d283" = 3.65
  dimension "d284" = 5
  dimension "d285" = 6.5
  dimension "d286" = 6.5
  dimension "d287" = 3
  dimension "d288" = 3
  dimension "d289" = 3
  dimension "d290" = 6.5
  dimension "d291" = 6.5
  dimension "d292" = 3.75
  dimension "d293" = 3.75
  dimension "d294" = 3.75
  dimension "d295" = 6.5
  dimension "d296" = 3.75
  dimension "d297" = 6.5
  dimension "d298" = 3.75
  dimension "d299" = 6.5
  dimension "d300" = 3.75
  dimension "d301" = 6.5
  dimension "d302" = 5
  dimension "d303" = 6.5
  measures "d245" distance of L37 P0
  measures "d246" distance of L1 P7
  measures "d247" distance of L1 L19
  measures "d248" distance of L17 P6
  measures "d249" distance of L21 L33
  measures "d250" distance of L33 P5
  measures "d251" distance of L23 P4
  measures "d252" distance of L7 P3
  measures "d253" distance of L15 P1
  measures "d254" distance of L31 P2
  measures "d255" distance of L25 P0
  measures "d256" distance of P29 L40
  measures "d257" distance of P29 L41
  measures "d258" distance of P28 L41
  measures "d259" distance of P27 L42
  measures "d260" distance of P26 L42
  measures "d261" distance of P25 L42
  measures "d262" distance of L43 L44
  measures "d263" distance of P25 L43
  measures "d264" distance of P26 L45
  measures "d265" distance of P27 L46
  measures "d266" distance of P28 L47
  measures "d267" distance of P29 L48
  measures "d268" distance of P9 L49
  measures "d269" distance of P9 L50
  measures "d270" distance of P10 L51
  measures "d271" distance of P10 L52
  measures "d272" distance of P10 L53
  measures "d273" distance of P9 L53
  measures "d274" distance of P11 L53
  measures "d275" distance of P11 L54
  measures "d276" distance of P12 L55
  measures "d277" distance of P12 L53
  measures "d278" distance of P13 L53
  measures "d279" distance of P13 L56
  measures "d280" distance of P14 L57
  measures "d281" distance of P14 L53
  measures "d282" distance of P15 L53
  measures "d283" distance of P15 L58
  measures "d284" distance of P16 L59
  measures "d285" distance of P16 L60
  measures "d286" distance of P17 L60
  measures "d287" distance of P17 L61
  measures "d288" distance of P18 L62
  measures "d289" distance of P18 L63
  measures "d290" distance of P18 L60
  measures "d291" distance of P19 L60
  measures "d292" distance of P19 L64
  measures "d293" distance of P19 L65
  measures "d294" distance of P20 L66
  measures "d295" distance of P20 L60
  measures "d296" distance of P21 L67
  measures "d297" distance of P21 L60
  measures "d298" distance of P22 L68
  measures "d299" distance of P22 L60
  measures "d300" distance of P23 L69
  measures "d301" distance of P23 L60
  measures "d302" distance of P24 L70
  measures "d303" distance of P24 L60